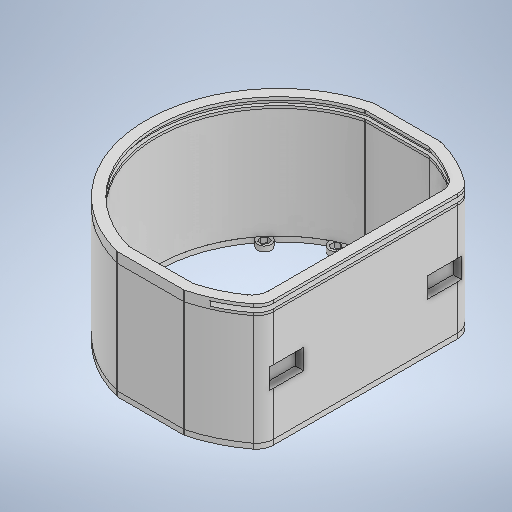
# Autodesk Inventor part: carcasa4.0
Saved by Autodesk Inventor 2025.3 (Build 293356030, 356C)
## iProperties
Created: 2025-08-27
Part Number: carcasa4.0
Material: Generic
Document SubType Name: Modeling
Designer: cdavi
Density: 1 g/cm^3
Appearance: Default
Author: cdavi
Autodesk Inventor part; units mm, degrees
ref_plane "YZ Plane" through (0, 0, 0) normal (1, 0, 0) x (0, 1, 0)
ref_plane "XZ Plane" through (0, 0, 0) normal (0, 1, 0) x (-1, 0, 0)
ref_plane "XY Plane" through (0, 0, 0) normal (0, 0, 1) x (1, 0, 0)
sketch "Sketch1" plane through (0, 0, 0) normal (0, 1, 0) x (-1, 0, 0)
  line L0 (18.5405, 69.5) -> (-18.5405, 69.5)
  line L1 (0, 0) -> (-51, 0) construction
  line L2 (19.3326, 75.5) -> (-19.3326, 75.5)
  line L3 (18.5405, -69.5) -> (-18.8082, -69.5)
  line L4 (19.3326, -75.5) -> (-19.3326, -75.5)
  line L5 (0, 0) -> (0, 75.5) construction
  line L6 (-45, 51.1762) -> (-45, -51.1762)
  line L7 (-51, 54.2494) -> (-51, -54.2494)
  arc A0 (-40.6452, -59.4304) -> (-18.8082, -69.5) centre (0, 0) ccw
  arc A1 (-47.0294, -62.2273) -> (-19.8414, -75.4342) centre (0, 0) ccw
  arc A2 (19.8414, -75.4342) -> (19.8414, 75.4342) centre (0, 0) ccw
  arc A3 (-19.8414, 75.4342) -> (-47.0294, 62.2273) centre (0, 0) ccw
  arc A4 (19.0702, -69.4286) -> (19.0702, 69.4286) centre (0, 0) ccw
  arc A5 (-19.0702, 69.4286) -> (-40.6452, 59.4304) centre (0, 0) ccw
  arc A6 (-19.8414, -75.4342) -> (-19.3326, -75.5) centre (-19.3326, -73.5) ccw
  arc A7 (19.3326, -75.5) -> (19.8414, -75.4342) centre (19.3326, -73.5) ccw
  arc A8 (18.5405, -69.5) -> (19.0702, -69.4286) centre (18.5405, -67.5) ccw
  arc A9 (19.0702, 69.4286) -> (18.5405, 69.5) centre (18.5405, 67.5) ccw
  arc A10 (19.8414, 75.4342) -> (19.3326, 75.5) centre (19.3326, 73.5) ccw
  arc A11 (-18.5405, 69.5) -> (-19.0702, 69.4286) centre (-18.5405, 67.5) ccw
  arc A12 (-19.3326, 75.5) -> (-19.8414, 75.4342) centre (-19.3326, 73.5) ccw
  arc A13 (-40.6452, 59.4304) -> (-45, 51.1762) centre (-35, 51.1762) ccw
  arc A14 (-47.0294, 62.2273) -> (-51, 54.2494) centre (-41, 54.2494) ccw
  arc A15 (-51, -54.2494) -> (-47.0294, -62.2273) centre (-41, -54.2494) ccw
  arc A16 (-45, -51.1762) -> (-40.6452, -59.4304) centre (-35, -51.1762) ccw
  point P0 (-19.5895, 75.5)
  point P1 (18.8082, -69.5)
  point P2 (19.5895, -75.5)
  point P3 (-19.5895, -75.5)
  point P4 (-51, -59.0169)
  point P5 (-45, 56.205)
  point P6 (-45, -56.205)
  point P7 (-51, 59.0169)
  point P8 (19.5895, 75.5)
  point P9 (18.8082, 69.5)
  point P10 (-18.8082, 69.5)
  dimension "d2" = 69.5
  dimension "d4" = 6
  dimension "d6" = 45
  dimension "d7" = 6
  dimension "d8" = 2
  dimension "d9" = 10
  dimension "d10" = 72
  dimension "d11" = 78
  dimension "d12" = 72
  dimension "d13" = 78
  constraints: 45 point on circle, 22 tangent, 17 centre point, 16 end point, 11 point on line, 9 equal radius, 4 symmetric about line, 3 vertical, 2 coincident, 2 horizontal, 2 midpoint, 1 parallel
  measures "d2" distance between parallel lines of L1 L0
  measures "d4" distance between parallel lines of L0 L2
  measures "d6" distance between parallel lines of L6 L5
  measures "d7" distance between parallel lines of L7 L6
  measures "d8" radius of A6
  measures "d9" radius of A13
  measures "d10" radius of A4
  measures "d11" radius of A2
  measures "d12" radius of A0
  measures "d13" radius of A1
extrude "Extrusion1" add sketch "Sketch1" along normal blind 65
sketch "Sketch2" plane through (51, 0, 54.2494) normal (1, 0, 0) x (0, 0, -1)
  line L0 (54.2494, 0) -> (54.2494, 65) construction
  line L1 (105.4256, 65) -> (3.0733, 65) projected
  line L2 (-2.1848, 38) -> (17.8152, 38)
  line L3 (17.8152, 38) -> (17.8152, 26)
  line L4 (17.8152, 26) -> (-2.1848, 26)
  line L5 (-2.1848, 26) -> (-2.1848, 38)
  line L6 (0, 0) -> (108.4988, 0) projected
  line L7 (-21.1848, 0) -> (-21.1848, 65) projected
  line L8 (110.6836, 38) -> (90.6836, 38)
  line L9 (90.6836, 38) -> (90.6836, 26)
  line L10 (90.6836, 26) -> (110.6836, 26)
  line L11 (110.6836, 26) -> (110.6836, 38)
  dimension "d16" = 26
  dimension "d17" = 19
  dimension "d18" = 12
  dimension "d19" = 20
  constraints: 18 end point, 4 symmetric about line, 2 parallel, 1 horizontal, 1 midpoint, 1 perpendicular
  measures "d16" distance between parallel lines of L6 L4
  measures "d17" distance between parallel lines of L5 L7
  measures "d18" distance of L2.end L3.end
  measures "d19" distance of L2.start L2.end
extrude "Extrusion2" cut sketch "Sketch2" against normal blind 5
sketch "Sketch3" plane through (51, 0, 54.2494) normal (1, 0, 0) x (0, 0, -1)
  line L0 (3.568, 49.2223) -> (17.7975, 43.9952) construction
  line L1 (2.8909, 47.379) -> (17.1204, 42.1519)
  line L2 (18.4746, 45.8385) -> (4.2452, 51.0656)
  arc A0 (4.2452, 51.0656) -> (2.8909, 47.379) centre (3.568, 49.2223) ccw
  arc A1 (17.1204, 42.1519) -> (18.4746, 45.8385) centre (17.7975, 43.9952) ccw
  arc A2 (44.4296, 11.624) -> (34.6921, 2.9774) centre (43.8866, 2.4292) ccw construction
  arc A3 (44.531, 13.3402) -> (32.9759, 3.0797) centre (43.8866, 2.4292) ccw
  arc A4 (44.3283, 9.9077) -> (36.4083, 2.8751) centre (43.8866, 2.4292) ccw
  arc A5 (44.3283, 9.9077) -> (44.531, 13.3402) centre (44.4296, 11.624) ccw
  arc A6 (32.9759, 3.0797) -> (36.4083, 2.8751) centre (34.6921, 2.9774) ccw
  line L3 (54.2494, 0) -> (54.2494, 65) construction
  line L4 (105.6079, 47.379) -> (91.3785, 42.1519)
  line L5 (90.0242, 45.8385) -> (104.2537, 51.0656)
  arc A7 (105.6079, 47.379) -> (104.2537, 51.0656) centre (104.9308, 49.2223) ccw
  arc A8 (90.0242, 45.8385) -> (91.3785, 42.1519) centre (90.7014, 43.9952) ccw
  point P0 (10.6828, 46.6088)
  constraints: 18 point on circle, 12 end point, 9 centre point, 8 tangent, 6 symmetric about line, 1 midpoint, 1 parallel, 2 other
extrude "Extrusion3" [suppressed]
extrude "Extrusion4" add sketch "Sketch1" along normal blind 3 from surface at 65 separate body contours A9 A4 A8 L3 A0 A16 L6 A13 A5 A11 L0 | A10 A2 A7 L4 A6 A1 A15 L7 A14 A3 A12 L2
sketch "Sketch5" plane through (-19.3326, 68, 75.5) normal (0, 1, 0) x (1, 0, 0)
  circle A0 centre (19.3326, 75.5) radius 8.5
  circle A1 centre (-10.6674, 75.5) radius 2.5
  line L0 (27.4567, 73) -> (36.3326, 73)
  line L1 (36.3326, 73) -> (36.3326, 78)
  line L2 (36.3326, 78) -> (27.4567, 78)
  line L3 (36.3326, 75.5) -> (70.3326, 75.5)
  line L4 (70.3326, 21.2506) -> (70.3326, 129.7494) projected
  line L5 (-10.6674, 75.5) -> (-58.6674, 75.5)
  arc A2 (-0.5088, 150.9342) -> (-0.5088, 0.0658) centre (19.3326, 75.5) ccw projected
  dimension "d26" = 17
  dimension "d27" = 5
  dimension "d31" = 5
  dimension "d32" = 17
  dimension "d47" = 30
  dimension "d204" = 34
  dimension "d205" = 48
  dimension "d206" = 51
  constraints: 10 end point, 3 point on circle, 2 centre point, 2 horizontal alignment, 2 midpoint, 2 perpendicular, 1 coincident, 1 horizontal, 1 point on line
  measures "d26" diameter of A0
  measures "d27" diameter of A1
  measures "d31" distance between parallel lines of L2 L0
  measures "d32" distance from line of A0.centre L1
  measures "d47" distance of A0.centre L5.start
  measures "d204" distance of L3.start L3.end
  measures "d205" distance of L5.start L5.end
  measures "d206" distance from line of L4 point (19.333, 75.5)
extrude "Extrusion5" cut sketch "Sketch5" against normal through all bodies 2
sketch "Sketch6" plane through (0, 0, 0) normal (0, 1, 0) x (-1, 0, 0)
  circle A0 centre (0, 0) radius 69 construction
  arc A1 (-19.0702, 69.4286) -> (-40.6452, 59.4304) centre (0, 0) ccw projected
  arc A2 (-40.6452, 59.4304) -> (-45, 51.1762) centre (-35, 51.1762) ccw projected
  line L0 (-45, -51.1762) -> (-45, 51.1762) projected
  arc A3 (-45, -51.1762) -> (-40.6452, -59.4304) centre (-35, -51.1762) ccw projected
  arc A4 (-40.6452, -59.4304) -> (-18.8082, -69.5) centre (0, 0) ccw projected
  line L1 (18.5405, -69.5) -> (-18.8082, -69.5) construction
  arc A5 (19.0702, -69.4286) -> (19.0702, 69.4286) centre (0, 0) ccw projected
  line L2 (-18.5405, 69.5) -> (18.5405, 69.5) construction
  line L3 (19.3326, 75.5) -> (-19.3326, 75.5) projected
  arc A6 (-19.8414, 75.4342) -> (-47.0294, 62.2273) centre (0, 0) ccw projected
  arc A7 (-47.0294, 62.2273) -> (-51, 54.2494) centre (-41, 54.2494) ccw projected
  line L4 (-51, 54.2494) -> (-51, -54.2494) projected
  arc A8 (-51, -54.2494) -> (-47.0294, -62.2273) centre (-41, -54.2494) ccw projected
  arc A9 (-47.0294, -62.2273) -> (-19.8414, -75.4342) centre (0, 0) ccw projected
  line L5 (-19.3326, -75.5) -> (19.3326, -75.5) projected
  arc A10 (19.8414, -75.4342) -> (19.8414, 75.4342) centre (0, 0) ccw projected
  arc A11 (-18.2665, 63.4219) -> (-37.2581, 54.4779) centre (0, 0) ccw construction
  arc A12 (-37.2581, 54.4779) -> (-39, 51.1762) centre (-35, 51.1762) ccw construction
  line L6 (-39, 51.1762) -> (-39, -51.1762) construction
  arc A13 (-39, -51.1762) -> (-37.2581, -54.4779) centre (-35, -51.1762) ccw construction
  arc A14 (-37.2581, -54.4779) -> (-18.2665, -63.4219) centre (0, 0) ccw construction
  line L7 (-17.713, -63.5) -> (17.713, -63.5) construction
  line L8 (-17.713, 63.5) -> (17.713, 63.5) construction
  arc A15 (18.2665, -63.4219) -> (18.2665, 63.4219) centre (0, 0) ccw construction
  arc A16 (-8.124, -2.5) -> (-8.124, 2.5) centre (0, 0) ccw projected
  line L9 (0, 0) -> (52.8571, 44.3523) construction
  line L10 (0, 0) -> (78, 0) construction
  circle A17 centre (52.8571, 44.3523) radius 2.85 construction
  line L11 (0, 0) -> (0, -69) construction
  circle A18 centre (29.1607, 62.5352) radius 2.85 construction
  line L12 (29.1607, 62.5352) -> (0, 0) construction
  circle A19 centre (-41.5, 20) radius 2.85 construction
  circle A20 centre (-29.1607, 62.5352) radius 2.85 construction
  line L13 (-29.1607, 62.5352) -> (0, 0) construction
  arc A21 (-17.713, 63.5) -> (-18.2665, 63.4219) centre (-17.713, 61.5) ccw construction
  arc A22 (-18.2665, -63.4219) -> (-17.713, -63.5) centre (-17.713, -61.5) ccw construction
  arc A23 (17.713, -63.5) -> (18.2665, -63.4219) centre (17.713, -61.5) ccw construction
  arc A24 (18.2665, 63.4219) -> (17.713, 63.5) centre (17.713, 61.5) ccw construction
  arc A25 (-19.8414, -75.4342) -> (-19.3326, -75.5) centre (-19.3326, -73.5) ccw projected
  arc A26 (19.3326, -75.5) -> (19.8414, -75.4342) centre (19.3326, -73.5) ccw projected
  arc A27 (19.8414, 75.4342) -> (19.3326, 75.5) centre (19.3326, 73.5) ccw projected
  arc A28 (-19.3326, 75.5) -> (-19.8414, 75.4342) centre (-19.3326, 73.5) ccw projected
  circle A29 centre (52.8571, -44.3523) radius 2.85 construction
  circle A30 centre (29.1607, -62.5352) radius 2.85 construction
  circle A31 centre (-41.5, -20) radius 2.85 construction
  circle A32 centre (-29.1607, -62.5352) radius 2.85 construction
  line L14 (19.0702, 63.1849) -> (19.0702, 69.4286)
  line L15 (-19.0702, 63.1849) -> (-19.0702, 69.4286)
  line L16 (19.0702, 69.4286) -> (-19.0702, 69.4286)
  line L17 (19.0702, -63.1849) -> (19.0702, -69.4286)
  line L18 (-19.0702, -63.1849) -> (-19.0702, -69.4286)
  line L19 (19.0702, -69.4286) -> (-19.0702, -69.4286)
  circle A33 centre (52.8571, 44.3523) radius 4
  circle A34 centre (29.1607, 62.5352) radius 4
  line L20 (50.0504, 43.8574) -> (51.0251, 46.5356)
  line L21 (51.0251, 46.5356) -> (53.8318, 47.0305)
  line L22 (53.8318, 47.0305) -> (55.6638, 44.8472)
  line L23 (55.6638, 44.8472) -> (54.689, 42.1691)
  line L24 (54.689, 42.1691) -> (51.8823, 41.6742)
  line L25 (51.8823, 41.6742) -> (50.0504, 43.8574)
  line L26 (26.8261, 60.9005) -> (26.5777, 63.7397)
  line L27 (26.5777, 63.7397) -> (28.9123, 65.3744)
  line L28 (28.9123, 65.3744) -> (31.4952, 64.1699)
  line L29 (31.4952, 64.1699) -> (31.7436, 61.3308)
  line L30 (31.7436, 61.3308) -> (29.4091, 59.6961)
  line L31 (29.4091, 59.6961) -> (26.8261, 60.9005)
  circle A35 centre (-41.5, 20) radius 4
  line L32 (-43.9682, 18.575) -> (-43.9682, 21.425)
  line L33 (-43.9682, 21.425) -> (-41.5, 22.85)
  line L34 (-41.5, 22.85) -> (-39.0318, 21.425)
  line L35 (-39.0318, 21.425) -> (-39.0318, 18.575)
  line L36 (-39.0318, 18.575) -> (-41.5, 17.15)
  line L37 (-41.5, 17.15) -> (-43.9682, 18.575)
  line L38 (-41.5, 24) -> (-45, 24)
  line L39 (-41.5, 16) -> (-45, 16)
  circle A36 centre (-29.1607, 62.5352) radius 4
  line L40 (-29.4091, 59.6961) -> (-31.7436, 61.3308)
  line L41 (-31.7436, 61.3308) -> (-31.4952, 64.1699)
  line L42 (-31.4952, 64.1699) -> (-28.9123, 65.3744)
  line L43 (-28.9123, 65.3744) -> (-26.5777, 63.7397)
  line L44 (-26.5777, 63.7397) -> (-26.8261, 60.9005)
  line L45 (-26.8261, 60.9005) -> (-29.4091, 59.6961)
  line L46 (-32.7354, 60.7404) -> (-34.082, 63.4225)
  circle A37 centre (52.8571, -44.3523) radius 4
  circle A38 centre (29.1607, -62.5352) radius 4
  circle A39 centre (-41.5, -20) radius 4
  line L47 (-41.5, -24) -> (-45, -24)
  line L48 (-41.5, -16) -> (-45, -16)
  circle A40 centre (-29.1607, -62.5352) radius 4
  line L49 (-32.7354, -60.7404) -> (-34.082, -63.4225)
  line L50 (50.0504, -43.8574) -> (51.0251, -46.5356)
  line L51 (51.0251, -46.5356) -> (53.8318, -47.0305)
  line L52 (53.8318, -47.0305) -> (55.6638, -44.8472)
  line L53 (55.6638, -44.8472) -> (54.689, -42.1691)
  line L54 (54.689, -42.1691) -> (51.8823, -41.6742)
  line L55 (51.8823, -41.6742) -> (50.0504, -43.8574)
  line L56 (26.8261, -60.9005) -> (26.5777, -63.7397)
  line L57 (26.5777, -63.7397) -> (28.9123, -65.3744)
  line L58 (28.9123, -65.3744) -> (31.4952, -64.1699)
  line L59 (31.4952, -64.1699) -> (31.7436, -61.3308)
  line L60 (31.7436, -61.3308) -> (29.4091, -59.6961)
  line L61 (29.4091, -59.6961) -> (26.8261, -60.9005)
  line L62 (-29.4091, -59.6961) -> (-31.7436, -61.3308)
  line L63 (-31.7436, -61.3308) -> (-31.4952, -64.1699)
  line L64 (-31.4952, -64.1699) -> (-28.9123, -65.3744)
  line L65 (-28.9123, -65.3744) -> (-26.5777, -63.7397)
  line L66 (-26.5777, -63.7397) -> (-26.8261, -60.9005)
  line L67 (-26.8261, -60.9005) -> (-29.4091, -59.6961)
  line L68 (-43.9682, -18.575) -> (-43.9682, -21.425)
  line L69 (-43.9682, -21.425) -> (-41.5, -22.85)
  line L70 (-41.5, -22.85) -> (-39.0318, -21.425)
  line L71 (-39.0318, -21.425) -> (-39.0318, -18.575)
  line L72 (-39.0318, -18.575) -> (-41.5, -17.15)
  line L73 (-41.5, -17.15) -> (-43.9682, -18.575)
  line L74 (50.1982, 47.3407) -> (52.4404, 49.3357)
  line L75 (55.3383, 41.2149) -> (57.6923, 43.0766)
  line L76 (32.7354, 60.7404) -> (34.082, 63.4225)
  line L77 (50.1982, -47.3407) -> (52.4404, -49.3357)
  line L78 (55.3383, -41.2149) -> (57.6923, -43.0766)
  line L79 (32.7354, -60.7404) -> (34.082, -63.4225)
  line L80 (-25.488, 64.1199) -> (-26.6769, 66.8756)
  line L81 (25.488, 64.1199) -> (26.6769, 66.8756)
  line L82 (-25.488, -64.1199) -> (-26.6769, -66.8756)
  line L83 (25.488, -64.1199) -> (26.6769, -66.8756)
  line L84 (-18.5405, 69.5) -> (-51, 69.5)
  line L85 (-51, 69.5) -> (-51, 54.2494)
  line L86 (-35.4083, 69.5) -> (-18.5405, 69.5)
  point P0 (-17.9931, -63.5)
  point P1 (-19.0702, 63.1849)
  point P2 (19.0702, -63.1849)
  point P3 (-19.0702, -63.1849)
  point P4 (29.1607, 62.5352)
  point P5 (-19.0702, -69.4286)
  point P6 (-34.082, -63.4225)
  point P7 (-45, -24)
  point P8 (-45, -16)
  point P9 (57.6923, -43.0766)
  point P10 (55.3383, -41.2149)
  point P11 (52.4404, -49.3357)
  point P12 (34.082, -63.4225)
  point P13 (-27.9581, 66.3502)
  point P14 (-27.9581, -66.3502)
  point P15 (27.9581, -66.3502)
  point P16 (27.9581, 66.3502)
  point P17 (-45, 21.9365)
  point P18 (-45, 18.0635)
  point P19 (-32.8561, 64.0662)
  point P20 (32.8561, -64.0662)
  point P21 (56.8533, -44.1781)
  point P22 (53.3794, -48.3181)
  point P23 (-32.8561, -64.0662)
  point P24 (-45, -21.9365)
  point P25 (-45, -18.0635)
  point P26 (53.3794, 48.3181)
  point P27 (56.8533, 44.1781)
  point P28 (32.8561, 64.0662)
  point P29 (25.488, -64.1199)
  point P30 (26.6769, -66.8756)
  point P31 (-26.6769, -66.8756)
  point P32 (-25.488, -64.1199)
  point P33 (34.0084, -67.0387)
  point P34 (-28.5882, -71.3052)
  point P35 (28.5882, -71.3052)
  point P36 (28.5882, 71.3052)
  point P37 (-28.5882, 71.3052)
  point P38 (34.0084, 67.0387)
  point P39 (-19.0702, -69.4286)
  point P40 (-34.0084, -67.0387)
  point P41 (-34.0084, 67.0387)
  dimension "d33" = 138
  dimension "d39" = 5.7
  dimension "d34" = 6
  dimension "d35" = 6
  dimension "d36" = 6
  dimension "d37" = 40
  dimension "d38" = 25
  dimension "d40" = 20
  dimension "d41" = 3.5
  dimension "d42" = 25
  dimension "d44" = 2
  dimension "d61" = 8
  dimension "d62" = 8
  dimension "d63" = 8
  dimension "d64" = 8
  dimension "d171" = 90
  dimension "d172" = 15.2506
  constraints: 162 end point, 52 symmetric about line, 38 point on circle, 20 centre point, 16 tangent, 10 coincident, 6 perpendicular, 4 point on line, 3 equal radius, 2 parallel, 2 vertical, 1 collinear, 1 horizontal, 93 other
  measures "d34" radial gap between concentric circles of A1 A11
  measures "d35" distance between parallel lines of L2 L8
  measures "d36" radial gap between concentric circles of A5 A15
  measures "d37" angle of L10 L9
  measures "d38" angle of L11 L12
  measures "d40" distance from line of point (-41.5, 20) L10
  measures "d41" distance from line of L0 point (-41.5, 20)
  measures "d42" angle of L11 L13
  measures "d44" radius of A21
  measures "d61" diameter of A33
  measures "d62" diameter of A34
  measures "d63" diameter of A35
  measures "d64" diameter of A36
  measures "d171" angle of L85 L84
  measures "d172" distance of L84.end L4.start
extrude "Extrusion6" add sketch "Sketch6" against normal blind 3 separate body contours L80 A36 A1 | A36 A1 | A1 A36 | A5 A34 L81 | A36 L46 A1 | A34 A5 | A5 A34 | A5 L76 A34 | A5 A33 L74 | L38 A35 L0 | A33 A5 | A5 A33 | A35 L0 | L0 A35 | A5 L75 A33 | A35 L39 L0 | A5 A37 L78 | L48 A39 L0 | A37 A5 | A5 A37 | A39 L0 | L0 A39 | A5 L77 A37 | A39 L47 L0 | A5 A38 L79 | A38 A5 | A5 A38 | A5 L83 A38 | L49 A40 A4 | A40 A4 | A4 A40 | A40 L82 A4 | A27 A10 A26 L5 A25 A9 A8 L4 A7 A6 A28 L3
sketch "Sketch14" plane through (0, 65, 0) normal (0, 1, 0) x (1, 0, 0)
  arc A0 (-19.8414, 75.4342) -> (-19.8414, -75.4342) centre (0, 0) ccw projected
  arc A1 (-19.8414, -75.4342) -> (-19.3326, -75.5) centre (-19.3326, -73.5) ccw projected
  line L0 (-19.3326, -75.5) -> (19.3326, -75.5) projected
  arc A2 (19.3326, -75.5) -> (19.8414, -75.4342) centre (19.3326, -73.5) ccw projected
  arc A3 (19.8414, -75.4342) -> (47.0294, -62.2273) centre (0, 0) ccw projected
  arc A4 (47.0294, -62.2273) -> (51, -54.2494) centre (41, -54.2494) ccw projected
  line L1 (51, -54.2494) -> (51, 54.2494) projected
  arc A5 (51, 54.2494) -> (47.0294, 62.2273) centre (41, 54.2494) ccw projected
  arc A6 (47.0294, 62.2273) -> (19.8414, 75.4342) centre (0, 0) ccw projected
  arc A7 (19.8414, 75.4342) -> (19.3326, 75.5) centre (19.3326, 73.5) ccw projected
  line L2 (19.3326, 75.5) -> (-19.3326, 75.5) projected
  arc A8 (-19.3326, 75.5) -> (-19.8414, 75.4342) centre (-19.3326, 73.5) ccw projected
  line L3 (-18.5405, 69.5) -> (18.8082, 69.5) projected
  arc A9 (40.6452, 59.4304) -> (18.8082, 69.5) centre (0, 0) ccw projected
  arc A10 (45, 51.1762) -> (40.6452, 59.4304) centre (35, 51.1762) ccw projected
  line L4 (45, 51.1762) -> (45, -51.1762) projected
  arc A11 (40.6452, -59.4304) -> (45, -51.1762) centre (35, -51.1762) ccw projected
  arc A12 (19.0702, -69.4286) -> (40.6452, -59.4304) centre (0, 0) ccw projected
  arc A13 (18.5405, -69.5) -> (19.0702, -69.4286) centre (18.5405, -67.5) ccw projected
  line L5 (18.5405, -69.5) -> (-18.5405, -69.5) projected
  arc A14 (-19.0702, -69.4286) -> (-18.5405, -69.5) centre (-18.5405, -67.5) ccw projected
  arc A15 (-19.0702, 69.4286) -> (-19.0702, -69.4286) centre (0, 0) ccw projected
  arc A16 (-18.5405, 69.5) -> (-19.0702, 69.4286) centre (-18.5405, 67.5) ccw projected
extrude "Extrusion11" add sketch "Sketch14" along normal blind 6 separate body
sketch "Sketch15" plane through (51, 65, 54.2494) normal (1, 0, 0) x (0, 0, -1)
  line L0 (54.2494, 6) -> (54.2494, 0)
  line L1 (54.2494, 6) -> (0, 6)
  line L2 (0, 6) -> (-17.251, 6)
  line L3 (-17.251, 6) -> (-17.251, 0)
  line L4 (-17.251, 0) -> (0, 0)
  line L5 (0, 0) -> (54.2494, 0)
  line L6 (3.0733, 0) -> (54.2494, 0)
  line L7 (54.2494, 6) -> (0, 6)
  line L8 (54.2494, 6) -> (54.2494, 4.5)
  line L9 (54.2494, 4.5) -> (0, 4.246)
  line L10 (0, 0) -> (0, 6) projected
  line L11 (54.2494, 0) -> (54.2494, 1.5)
  line L12 (54.2494, 1.5) -> (0, 1.5)
  arc A0 (54.2494, 4.5) -> (54.2494, 4.5) centre (53.5042, 163.6577) ccw
  line L13 (0, 4.246) -> (-17.251, 4.246)
  line L14 (0, 1.5) -> (-17.251, 1.5)
  line L15 (54.2494, 6) -> (108.4988, 6)
  line L16 (108.4988, 6) -> (125.7498, 6)
  line L17 (125.7498, 6) -> (125.7498, 0)
  line L18 (125.7498, 0) -> (108.4988, 0)
  line L19 (108.4988, 0) -> (54.2494, 0)
  line L20 (105.4256, 0) -> (54.2494, 0)
  line L21 (54.2494, 6) -> (108.4988, 6)
  line L22 (54.2494, 4.5) -> (108.4988, 4.246)
  line L23 (108.4988, 0) -> (108.4988, 6)
  line L24 (54.2494, 1.5) -> (108.4988, 1.5)
  arc A1 (54.2494, 4.5) -> (54.2494, 4.5) centre (54.9946, 163.6577) ccw
  line L25 (108.4988, 4.246) -> (125.7498, 4.246)
  line L26 (108.4988, 1.5) -> (125.7498, 1.5)
  point P0 (54.2494, -65)
  dimension "d173" = 17.251
  dimension "d176" = 1.5
  dimension "d177" = 1.5
  dimension "d202" = 2.746
  constraints: 52 end point, 15 point on line, 11 symmetric about line, 6 perpendicular, 4 point on circle, 2 centre point, 1 collinear, 1 tangent, 1 other
  measures "d173" distance of L1.end L2.end
  measures "d176" distance of L0.start L8.end
  measures "d177" distance of L0.end L11.end
  measures "d202" distance between parallel lines of L14 L13
extrude "Extrusion12" cut sketch "Sketch15" against normal blind 70.071 contours L22 L23 L24 L0 | L0 L12 L10 L9 | L10 L14 L3 L13 | L25 L17 L26 L23 bodies 4
ref_plane "Work Plane1" through (0, 66.5, 0) normal (0, -1, 0) x (1, 0, 0)
sketch "Sketch18" plane through (0, 66.5, 0) normal (0, -1, 0) x (1, 0, 0)
  arc A0 (18.8082, -69.5) -> (40.6452, -59.4304) centre (0, 0) ccw projected
  arc A1 (-19.071, 69.4284) -> (-19.071, -69.4284) centre (0, 0) ccw
  arc A2 (-19.071, 71.5003) -> (-19.071, -71.5003) centre (0, 0) ccw
  line L0 (-19.071, 69.4284) -> (-19.071, 71.5003)
  line L1 (-19.071, -69.4284) -> (-19.071, -71.5003)
  point P0 (-19.0702, 69.4286)
  point P1 (-19.071, -71.5004)
  dimension "d209" = 148
  dimension "d211" = 72
  constraints: 5 point on circle, 4 end point, 2 centre point, 2 vertical, 1 coincident
  measures "d209" diameter of A2
  measures "d211" radius of A1
extrude "Extrusion14" cut sketch "Sketch18" against normal blind 2.746 bodies 4
body "Solid1"
body "Solid2"
body "Solid3"
body "Solid4"
